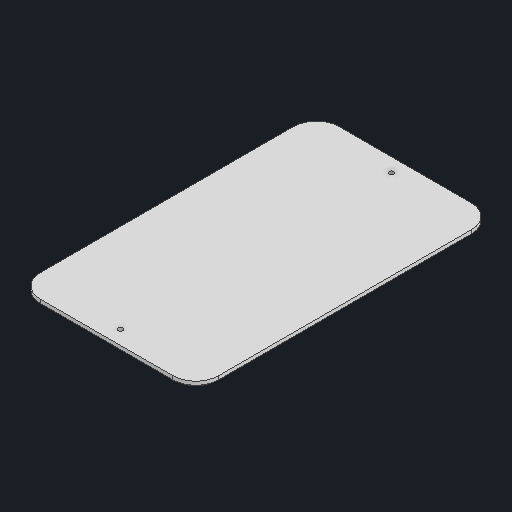
# Autodesk Inventor part: case5
Saved by Autodesk Inventor 2026.2 (Build 302298000, 298)
## iProperties
Created: 2026-02-03
Part Number: case5
Material: Generic
Document SubType Name: Modeling
Designer: mi
Density: 1 g/cm^3
Appearance: Default
Author: mi
## iProperties of the stored document case5_3DPrint.ipt
Created: 2026-02-04
Part Number: case5_3DPrint
Material: Generic
Document SubType Name: Modeling
Designer: mi
Density: 1 g/cm^3
Appearance: Default
Author: mi
Autodesk Inventor part; units mm, degrees
ref_plane "YZ Plane" through (0, 0, 0) normal (1, 0, 0) x (0, 1, 0)
ref_plane "XZ Plane" through (0, 0, 0) normal (0, 1, 0) x (-1, 0, 0)
ref_plane "XY Plane" through (0, 0, 0) normal (0, 0, 1) x (1, 0, 0)
sketch "Sketch1" plane through (0, 0, 0) normal (0, 1, 0) x (-1, 0, 0)
  line L0 (0, 0) -> (148, 0)
  line L1 (148, 0) -> (148, -248)
  line L2 (148, -248) -> (0, -248)
  line L3 (0, -248) -> (0, 0)
  dimension "d0" = 148
  dimension "d1" = 248
  constraints: 8 end point, 2 parallel, 1 horizontal, 1 perpendicular
  measures "d0" distance of L1.end L2.end
  measures "d1" distance of L0.end L1.end
extrude "Extrusion1" add sketch "Sketch1" along normal blind 3
fillet "Fillet1" radius 19 4 edges at (0, 1.5, 0) (-148, 1.5, 0) (0, 1.5, -248) (-148, 1.5, -248)
sketch "Sketch2" plane through (0, 0, 0) normal (0, -1, 0) x (1, 0, 0)
  arc A0 (-148, -229) -> (-129, -248) centre (-129, -229) ccw projected
  line L0 (-19, -248) -> (-129, -248) projected
  arc A1 (-19, -248) -> (0, -229) centre (-19, -229) ccw projected
  line L1 (0, -19) -> (0, -229) projected
  arc A2 (0, -19) -> (-19, 0) centre (-19, -19) ccw projected
  line L2 (-129, 0) -> (-19, 0) projected
  arc A3 (-129, 0) -> (-148, -19) centre (-129, -19) ccw projected
  line L3 (-148, -229) -> (-148, -19) projected
  arc A4 (-129, -5) -> (-143, -19) centre (-129, -19) ccw
  line L4 (-129, -5) -> (-19, -5)
  arc A5 (-5, -19) -> (-19, -5) centre (-19, -19) ccw
  line L5 (-5, -19) -> (-5, -229)
  arc A6 (-19, -243) -> (-5, -229) centre (-19, -229) ccw
  line L6 (-19, -243) -> (-129, -243)
  arc A7 (-143, -229) -> (-129, -243) centre (-129, -229) ccw
  line L7 (-143, -229) -> (-143, -19)
  line L8 (-63.5, -243) -> (-84.5, -243)
  line L9 (-84.5, -243) -> (-84.5, -227)
  line L10 (-84.5, -227) -> (-63.5, -227)
  line L11 (-63.5, -227) -> (-63.5, -243)
  line L12 (-143, -124) -> (-5, -124) construction
  line L13 (-63.5, -5) -> (-84.5, -5)
  line L14 (-84.5, -5) -> (-84.5, -21)
  line L15 (-84.5, -21) -> (-63.5, -21)
  line L16 (-63.5, -21) -> (-63.5, -5)
  circle A8 centre (-74, -11.5) radius 2
  line L17 (-74, -227) -> (-74, -21) construction
  circle A9 centre (-74, -236.5) radius 2
  point P0 (0, 0)
  point P1 (-74, -243)
  point P2 (-74, -5)
  point P3 (-84.5, -243)
  point P4 (-63.5, -5)
  point P5 (-84.5, -5)
  dimension "d12" = 21
  dimension "d13" = 21
  dimension "d14" = 5
  dimension "d16" = 4
  dimension "d18" = 225
  constraints: 28 end point, 8 point on circle, 6 centre point, 6 midpoint, 6 symmetric about line, 2 parallel, 2 point on line, 1 horizontal, 1 perpendicular, 8 other
  measures "d12" distance between parallel lines of L11 L9
  measures "d13" distance between parallel lines of L0 L10
  measures "d14" distance between parallel lines of L0 L6
  measures "d16" diameter of A8
  measures "d18" distance of A9.centre A8.centre
extrude "Extrusion2" add sketch "Sketch2" along normal blind 4 contours L4 L14 L15 L16 A5 L5 A6 L6 L11 L10 L9 A7 L7 A4
extrude "Extrusion4" cut sketch "Sketch2" against normal up to surface (3 mm away) contours A8 | A9
fillet "Fillet2" radius 4 4 edges at (-84.5, -2, -243) (-63.5, -2, -243) (-84.5, -2, -5) (-63.5, -2, -5)
equation "\"d5\" = d16"
equation "\"d19\" = d16"
body "Solid1"
